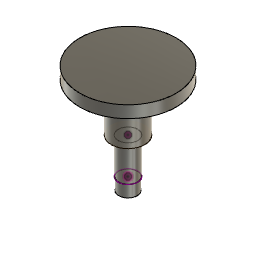
Secondary Pinion (Autodesk Fusion 360 design; units mm, degrees)
Autodesk Fusion 360 part; units mm, degrees
sketch "Sketch1" plane through (0, 0, 0) normal (0, 0, 1) x (1, 0, 0)
  circle A0 centre (0, 0) radius 7
  circle A1 centre (0, 0) radius 20
  dimension "d8" = 14
  dimension "d58" = 40
  constraint coincident A0.centre A1.centre
  measures "d8" diameter of A0
  measures "d58" diameter of A1
extrude "Extrude12" add sketch "Sketch1" along normal blind 5 makes body 1
extrude "Extrude2" add sketch "Sketch1" against normal blind 20 separate body contours A0 makes body 2
extrude "Extrude1" add sketch "Sketch1" against normal blind 20 separate body contours A0 makes body 3
sketch "Sketch3" plane through (0, 0, -20) normal (0, 0, -1) x (1, 0, 0)
  circle A0 centre (0, 0) radius 7
  circle A1 centre (0, 0) radius 4.05
  dimension "d31" = 8.1
  constraint coincident A0.centre A1.centre
  measures "d31" diameter of A1
extrude "Extrude6" add sketch "Sketch3" along normal blind 15 contours A1 bodies 2 3
sketch "Sketch6" plane through (0, 0, -35) normal (0, 0, -1) x (1, 0, 0)
  circle A0 centre (0, 0) radius 3.85
  circle A1 centre (0, 0) radius 4.05
  dimension "d47" = 7.7
  constraint coincident A0.centre A1.centre
  measures "d47" diameter of A0
extrude "Extrude9" add sketch "Sketch6" along normal blind 5 contours A0 bodies 2
delete_face "DeleteFace1" 1 faces at (6.9913, -0.3489, 3.3333) on bodies 1
equation "lower_part_outer_radius = 7 mm"
equation "lower_part_length = 20 mm"
equation "upper_part_outer_radius = 3.85 mm"
equation "upper_part_length = 5 mm"
equation "d8 = lower_part_outer_radius * 2"
equation "extra = 100 mm"
equation "d11 = -lower_part_length"
equation "d14 = -lower_part_length"
equation "d31 = bearing_part_outer_radius * 2"
equation "d32 = bearing_part_length"
equation "bearing_part_outer_radius = 4.05 mm"
equation "bearing_part_length = 15 mm"
equation "d47 = upper_part_outer_radius * 2"
equation "d48 = upper_part_length"
equation "base_part_outer_radius = 20 mm"
equation "base_part_length = 5 mm"
equation "d58 = base_part_outer_radius * 2"
equation "d59 = base_part_length"
